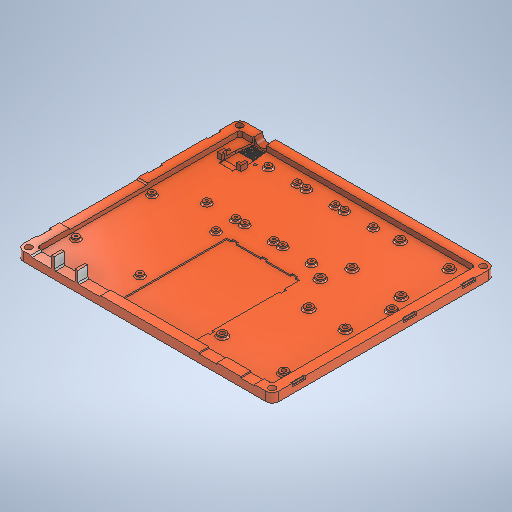
# Autodesk Inventor part: Electronic Base 5
Saved by Autodesk Inventor 2025.2 (Build 292293000, 293)
## iProperties
Created: 2025-02-05
Part Number: Electronic Base 5
Material: Generic
Document SubType Name: Modeling
Designer: caomi
Density: 1 g/cm^3
Appearance: Default
Author: caomi
Autodesk Inventor part; units mm, degrees
ref_plane "YZ Plane" through (0, 0, 0) normal (1, 0, 0) x (0, 1, 0)
ref_plane "XZ Plane" through (0, 0, 0) normal (0, 1, 0) x (-1, 0, 0)
ref_plane "XY Plane" through (0, 0, 0) normal (0, 0, 1) x (1, 0, 0)
sketch "Sketch1" plane through (0, 0, 0) normal (0, 1, 0) x (-1, 0, 0)
  line L0 (195, 170) -> (0, 170)
  line L1 (0, 170) -> (0, 0)
  line L2 (0, 0) -> (195, 0)
  line L3 (195, 0) -> (195, 170)
  line L4 (185.5, 76.5) -> (129.5, 76.5) construction
  line L5 (129.5, 76.5) -> (129.5, 161.5) construction
  line L6 (129.5, 161.5) -> (185.5, 161.5) construction
  line L7 (185.5, 161.5) -> (185.5, 76.5) construction
  circle A0 centre (182, 80) radius 0.9
  circle A1 centre (182, 138) radius 0.9
  circle A2 centre (133, 80) radius 0.9
  circle A3 centre (133, 138) radius 0.9
  line L8 (0, 0) -> (-136.9444, 0) construction
  line L9 (0, 0) -> (0, -49.9102) construction
  circle A4 centre (182, 80) radius 2.4
  circle A5 centre (182, 138) radius 2.4
  circle A6 centre (133, 80) radius 2.4
  circle A7 centre (133, 138) radius 2.4
  line L10 (187.5, 7.5) -> (7.5, 7.5)
  line L11 (7.5, 7.5) -> (7.5, 162.5)
  line L12 (7.5, 162.5) -> (187.5, 162.5)
  line L13 (187.5, 162.5) -> (187.5, 7.5)
  line L14 (64.5, 59.9) -> (11.16, 59.9) construction
  line L15 (11.16, 59.9) -> (11.16, 161.5) construction
  line L16 (11.16, 161.5) -> (64.5, 161.5) construction
  line L17 (64.5, 161.5) -> (64.5, 59.9) construction
  circle A8 centre (61.96, 71.33) radius 3.05
  circle A9 centre (61.96, 71.33) radius 1.55
  circle A10 centre (46.72, 95.46) radius 3.05
  circle A11 centre (46.72, 95.46) radius 1.55
  circle A12 centre (61.96, 146.26) radius 1.55
  circle A13 centre (18.78, 95.46) radius 3.05
  circle A14 centre (61.96, 146.26) radius 3.05
  circle A15 centre (18.78, 95.46) radius 1.55
  circle A16 centre (13.7, 64.98) radius 3.05
  circle A17 centre (13.7, 64.98) radius 1.55
  circle A18 centre (13.7, 147.53) radius 3.05
  circle A19 centre (13.7, 147.53) radius 1.55
  line L18 (124.5, 80.32) -> (69.75, 80.32) construction
  line L19 (69.75, 80.32) -> (69.75, 162) construction
  line L20 (69.75, 162) -> (124.5, 162) construction
  line L21 (124.5, 162) -> (124.5, 80.32) construction
  line L22 (59.33, 12.5) -> (16.33, 12.5) construction
  line L23 (16.33, 12.5) -> (16.33, 55.5) construction
  line L24 (16.33, 55.5) -> (59.33, 55.5) construction
  line L25 (59.33, 55.5) -> (59.33, 12.5) construction
  line L26 (157.5, 66.5) -> (131.5, 66.5) construction
  line L27 (131.5, 66.5) -> (131.5, 15.5) construction
  line L28 (131.5, 15.5) -> (157.5, 15.5) construction
  line L29 (157.5, 15.5) -> (157.5, 66.5) construction
  circle A20 centre (155.5, 17.5) radius 0.9
  circle A21 centre (155.5, 17.5) radius 2.4
  circle A22 centre (133.5, 17.5) radius 2.4
  circle A23 centre (133.5, 17.5) radius 0.9
  circle A24 centre (155.5, 64.5) radius 2.4
  circle A25 centre (155.5, 64.5) radius 0.9
  circle A26 centre (133.5, 64.5) radius 0.9
  circle A27 centre (133.5, 64.5) radius 2.4
  line L30 (102.5, 15.5) -> (128.5, 15.5) construction
  circle A28 centre (104.5, 17.5) radius 0.9
  circle A29 centre (126.5, 17.5) radius 0.9
  circle A30 centre (104.5, 17.5) radius 2.4
  circle A31 centre (126.5, 17.5) radius 2.4
  circle A32 centre (104.5, 64.5) radius 0.9
  circle A33 centre (104.5, 64.5) radius 2.4
  line L31 (102.5, 66.5) -> (102.5, 15.5) construction
  line L32 (128.5, 66.5) -> (102.5, 66.5) construction
  circle A34 centre (126.5, 64.5) radius 2.4
  line L33 (128.5, 15.5) -> (128.5, 66.5) construction
  circle A35 centre (126.5, 64.5) radius 0.9
  line L34 (73.5, 15.5) -> (99.5, 15.5) construction
  circle A36 centre (75.5, 17.5) radius 0.9
  circle A37 centre (97.5, 17.5) radius 0.9
  circle A38 centre (75.5, 17.5) radius 2.4
  circle A39 centre (97.5, 17.5) radius 2.4
  circle A40 centre (75.5, 64.5) radius 0.9
  circle A41 centre (75.5, 64.5) radius 2.4
  line L35 (73.5, 66.5) -> (73.5, 15.5) construction
  line L36 (99.5, 66.5) -> (73.5, 66.5) construction
  circle A42 centre (97.5, 64.5) radius 2.4
  line L37 (99.5, 15.5) -> (99.5, 66.5) construction
  circle A43 centre (97.5, 64.5) radius 0.9
  line L38 (69.25, 79.82) -> (125, 79.82)
  line L39 (125, 79.82) -> (125, 162.5)
  line L40 (125, 162.5) -> (69.25, 162.5)
  line L41 (69.25, 162.5) -> (69.25, 79.82)
  line L42 (99.125, 79.82) -> (95.125, 79.82)
  line L43 (95.125, 79.82) -> (95.125, 78.32)
  line L44 (95.125, 78.32) -> (99.125, 78.32)
  line L45 (99.125, 78.32) -> (99.125, 79.82)
  line L46 (117.825, 78.32) -> (121.825, 78.32)
  line L47 (121.825, 78.32) -> (121.825, 79.82)
  line L48 (117.825, 79.82) -> (117.825, 78.32)
  line L49 (72.425, 78.32) -> (76.425, 78.32)
  line L50 (76.425, 78.32) -> (76.425, 79.82)
  line L51 (72.425, 79.82) -> (72.425, 78.32)
  line L52 (69.25, 146.1) -> (67.75, 146.1)
  line L53 (67.75, 146.1) -> (67.75, 150.1)
  line L54 (67.75, 150.1) -> (69.25, 150.1)
  line L55 (69.25, 150.1) -> (69.25, 146.1)
  line L56 (69.25, 91.57) -> (67.75, 91.57)
  line L57 (67.75, 91.57) -> (67.75, 95.57)
  line L58 (67.75, 95.57) -> (69.25, 95.57)
  circle A44 centre (19.201, 15.82) radius 1.4
  circle A45 centre (19.201, 15.82) radius 2.9
  circle A46 centre (56.574, 15.82) radius 2.9
  circle A47 centre (56.574, 15.82) radius 1.4
  circle A48 centre (19.201, 52.557) radius 1.4
  circle A49 centre (19.201, 52.557) radius 2.9
  circle A50 centre (56.574, 52.557) radius 2.9
  circle A51 centre (56.574, 52.557) radius 1.4
  line L59 (144.5, 15.5) -> (144.5, 27.2667) construction
  line L60 (37.83, 12.5) -> (37.83, 30.4) construction
  line L61 (37.83, 59.9) -> (37.83, 76.07) construction
  point P0 (185.5, 119)
  point P1 (11.16, 110.7)
  point P2 (1.5544, 63)
  point P3 (2.0056, 63)
  point P4 (82.8344, 63)
  point P5 (83.2856, 63)
  point P6 (37.83, 161.5)
  point P7 (97.125, 78.32)
  point P8 (97.125, 79.82)
  point P9 (119.825, 78.32)
  point P10 (74.425, 78.32)
  point P11 (67.75, 148.1)
  point P12 (67.75, 93.57)
  point P13 (72.425, 79.82)
  point P14 (76.425, 79.82)
  point P15 (95.125, 79.82)
  dimension "d10" = 1.8
  dimension "d49" = 53.34
  dimension "d59" = 7.5
  dimension "d62" = 3.1
  dimension "d63" = 1.5
  dimension "d73" = 7.5
  dimension "d79" = 7.5
  dimension "d82" = 2.54
  dimension "d83" = 15.24
  dimension "d84" = 90.17
  dimension "d85" = 96.52
  dimension "d86" = 50.8
  dimension "d87" = 66.04
  dimension "d88" = 17.78
  dimension "d89" = 45.72
  dimension "d90" = 13.97
  dimension "d91" = 85
  dimension "d92" = 58
  dimension "d95" = 1.5
  dimension "d96" = 3.5
  dimension "d97" = 3.5
  dimension "d98" = 3.5
  dimension "d99" = 56
  dimension "d102" = 7.5
  dimension "d103" = 65
  dimension "d121" = 54.75
  dimension "d122" = 81.68
  dimension "d123" = 1
  dimension "d124" = 43
  dimension "d131" = 51
  dimension "d134" = 101.6
  dimension "d135" = 26
  dimension "d141" = 49
  dimension "d144" = 29
  dimension "d149" = 0.5
  dimension "d150" = 4
  dimension "d151" = 1.5
  dimension "d154" = 22.7
  dimension "d160" = 11.9
  dimension "d165" = 54.53
  dimension "d172" = 30
  dimension "d173" = 8
  dimension "d174" = 2
  dimension "d176" = 2.8
  dimension "d178" = 5
  dimension "d179" = 3.32
  dimension "d180" = 2.871
  dimension "d181" = 40.244
  dimension "d182" = 40.057
  dimension "d278" = 1.5
  dimension "d279" = 2
  dimension "d280" = 2
  dimension "d281" = 1.8
  dimension "d282" = 4.8
  dimension "d298" = 155
  dimension "d299" = 4.5
  dimension "d305" = 180
  constraints: 124 end point, 52 centre point, 26 equal radius, 21 coincident, 20 parallel, 13 perpendicular, 12 horizontal, 10 midpoint, 9 vertical alignment, 7 horizontal alignment, 5 vertical, 4 collinear, 3 point on line, 1 symmetric about line, 74 other
  measures "d10" diameter of A0
  measures "d49" distance of L15.end L16.end
  measures "d59" distance between parallel lines of L13 L3
  measures "d62" diameter of A9
  measures "d63" radial gap between concentric circles of A8 A9
  measures "d73" distance between parallel lines of L0 L12
  measures "d79" distance between parallel lines of L2 L10
  measures "d82" distance from line of L17 A12.centre
  measures "d83" distance from line of L16 A12.centre
  measures "d84" distance from line of L16 A9.centre
  measures "d85" distance from line of L16 A16.centre
  measures "d86" distance from line of L17 A17.centre
  measures "d87" distance from line of L16 A10.centre
  measures "d88" distance from line of L17 A10.centre
  measures "d89" distance from line of L17 A15.centre
  measures "d90" distance from line of L16 A18.centre
  measures "d91" distance of L4.end L5.end
  measures "d92" distance of A3.centre A2.centre
  measures "d95" radial gap between concentric circles of A4 A0
  measures "d96" distance from line of L4 A2.centre
  measures "d97" distance from line of L7 A0.centre
  measures "d98" distance from line of L5 A2.centre
  measures "d99" distance between parallel lines of L7 L5
  measures "d102" distance between parallel lines of L1 L11
  measures "d103" distance between parallel lines of L17 L5
  measures "d121" distance of L19.end L20.end
  measures "d122" distance of L18.end L19.end
  measures "d123" distance between parallel lines of L12 L16
  measures "d124" distance of L22.end L23.end
  measures "d131" distance of L28.end L26.start
  measures "d134" distance of L14.end L15.end
  measures "d135" distance of L27.end L28.end
  measures "d141" distance from line of L28 A24.centre
  measures "d144" distance of A22.centre A30.centre
  measures "d149" distance between parallel lines of L19 L41
  measures "d150" distance of L43.end L44.end
  measures "d151" distance between parallel lines of L38 L44
  measures "d154" distance of point (97.125, 78.32) point (119.825, 78.32)
  measures "d160" distance between parallel lines of L20 L54
  measures "d165" distance of L52.start L56.start
  measures "d172" distance between parallel lines of L13 L29
  measures "d173" distance between parallel lines of L10 L28
  measures "d174" distance between parallel lines of L7 L13
  measures "d176" diameter of A44
  measures "d178" vertical distance of L10.end L22.end
  measures "d179" distance from line of L22 A44.centre
  measures "d180" distance from line of L23 A44.centre
  measures "d181" distance from line of L23 A46.centre
  measures "d182" distance from line of L22 A48.centre
  measures "d278" radial gap between concentric circles of A44 A45
  measures "d279" distance from line of A21.centre L29
  measures "d280" distance from line of A20.centre L28
  measures "d281" diameter of A20
  measures "d282" diameter of A21
  measures "d298" distance of L10.end L11.end
  measures "d299" distance between parallel lines of L5 L39
  measures "d305" distance of L11.end L12.end
extrude "Base" add sketch "Sketch1" against normal blind 3 contours L3 L2 L1 L0 | A0 | A1 | A2 | A3 | A4 | A5 | A6 | A7 | L10 L11 L12 L41 L54 L53 L52 L58 L57 L56 L38 L51 L49 L50 L43 L44 L45 L48 L46 L47 L39 L13 | L39 L38 L41 L12 | L41 L52 L53 L54 | L47 L46 L48 L38 | L41 L56 L57 L58 | L45 L44 L43 L38 | L50 L49 L51 L38 | A8 | A9 | A10 | A11 | A12 | A13 | A14 | A15 | A16 | A17 | A18 | A19 | A20 | A21 | A22 | A23 | A24 | A25 | A26 | A27 | A28 | A29 | A30 | A31 | A32 | A33 | A34 | A35 | A36 | A37 | A38 | A39 | A40 | A41 | A42 | A43 | A44 | A45 | A46 | A47 | A48 | A49 | A50 | A51
extrude "Wall" add sketch "Sketch1" along normal blind 4 contours L3 L2 L1 L0
extrude "Breadboard Slot" cut sketch "Sketch1" against normal blind 1 contours L39 L38 L41 L12 | L41 L52 L53 L54 | L47 L46 L48 L38 | L41 L56 L57 L58 | L45 L44 L43 L38 | L50 L49 L51 L38
extrude "Electronic Mounting Holes" add sketch "Sketch1" along normal blind 2 contours A4 | A5 | A6 | A7 | A8 | A10 | A13 | A14 | A16 | A18 | A21 | A22 | A24 | A27 | A30 | A31 | A33 | A34 | A38 | A39 | A41 | A42 | A45 | A46 | A49 | A50
extrude "Deeper Mounting Holes" cut sketch "Sketch1" against normal blind 2 contours A0 | A1 | A2 | A3 | A9 | A11 | A12 | A15 | A17 | A19 | A20 | A23 | A25 | A26 | A28 | A29 | A32 | A35 | A36 | A37 | A40 | A43 | A44 | A47 | A48 | A51
chamfer "Chamfer2" distance 1 angle 45 26 edges at (-153.1, 0, 17.5) (-131.1, 0, 17.5) (-124.1, 0, 17.5) (-102.1, 0, 17.5) (-95.1, 0, 17.5) (-73.1, 0, 17.5) (-53.674, 0, 15.82) (-16.301, 0, 15.82) (-16.301, 0, 52.557) (-10.65, 0, 64.98) (-53.674, 0, 52.557) (-58.91, 0, 71.33) (-73.1, 0, 64.5) (-95.1, 0, 64.5) (-102.1, 0, 64.5) (-124.1, 0, 64.5) (-131.1, 0, 64.5) (-153.1, 0, 64.5) (-130.6, 0, 80) (-179.6, 0, 80) (-179.6, 0, 138) (-130.6, 0, 138) (-43.67, 0, 95.46) (-15.73, 0, 95.46) (-10.65, 0, 147.53) (-58.91, 0, 146.26)
fillet "Fillet1" radius 5 4 edges at (-195, 0.5, 0) (0, 0.5, 170) (-195, 0.5, 170) (0, 0.5, 0)
fillet "Fillet3" radius 2 4 edges at (-187.5, 2, 162.5) (-187.5, 2, 7.5) (-7.5, 2, 162.5) (-7.5, 2, 7.5)
sketch "Sketch2" plane through (0, 4, 0) normal (0, 1, 0) x (1, 0, 0)
  line L0 (-190, -170) -> (-5, -170) projected
  line L1 (-7.5, -162.5) -> (-187.5, -162.5) projected
  line L2 (-184.5, -162.5) -> (-168.5, -162.5)
  line L3 (-168.5, -162.5) -> (-168.5, -170)
  line L4 (-168.5, -170) -> (-184.5, -170)
  line L5 (-184.5, -170) -> (-184.5, -162.5)
  line L6 (-166.5, -162.5) -> (-150.5, -162.5)
  line L7 (-150.5, -162.5) -> (-150.5, -170)
  line L8 (-150.5, -170) -> (-166.5, -170)
  line L9 (-166.5, -170) -> (-166.5, -162.5)
  line L10 (-148.5, -162.5) -> (-131, -162.5)
  line L11 (-131, -162.5) -> (-131, -170)
  line L12 (-131, -170) -> (-148.5, -170)
  line L13 (-148.5, -170) -> (-148.5, -162.5)
  line L14 (-56, -162.5) -> (-42.36, -162.5)
  line L15 (-42.36, -162.5) -> (-42.36, -170)
  line L16 (-42.36, -170) -> (-56, -170)
  line L17 (-56, -170) -> (-56, -162.5)
  line L18 (-185.5, -161.5) -> (-185.5, -76.5) construction
  line L19 (-64.5, -161.5) -> (-64.5, -59.9) construction
  line L20 (-24, -162.5) -> (-13.67, -162.5)
  line L21 (-13.67, -162.5) -> (-13.67, -170)
  line L22 (-13.67, -170) -> (-24, -170)
  line L23 (-24, -170) -> (-24, -162.5)
  line L24 (-195, -5) -> (-195, -165) projected
  line L25 (-187.5, -9.5) -> (-187.5, -160.5) projected
  line L26 (-195, -137.5) -> (-187.5, -137.5)
  line L27 (-187.5, -137.5) -> (-187.5, -77.5)
  line L28 (-187.5, -77.5) -> (-195, -77.5)
  line L29 (-195, -77.5) -> (-195, -137.5)
  point P0 (0, 0)
  point P1 (-150.5, -162.5)
  point P2 (-168.5, -162.5)
  point P3 (-13.67, -166.25)
  point P4 (-56, -170)
  point P5 (-195, -77.5)
  point P6 (-187.5, -137.5)
  dimension "d104" = 16
  dimension "d107" = 16
  dimension "d109" = 17.5
  dimension "d113" = 13.64
  dimension "d114" = 1
  dimension "d115" = 19
  dimension "d116" = 37
  dimension "d117" = 8.5
  dimension "d118" = 40.5
  dimension "d119" = 10.33
  dimension "d300" = 25
  dimension "d301" = 85
  constraints: 48 end point, 12 parallel, 12 point on line, 6 horizontal, 6 perpendicular, 1 midpoint
  measures "d104" distance of L3.end L4.end
  measures "d107" distance of L7.end L8.end
  measures "d109" distance between parallel lines of L11 L13
  measures "d113" distance between parallel lines of L15 L17
  measures "d114" distance between parallel lines of L18 L5
  measures "d115" distance between parallel lines of L18 L9
  measures "d116" distance between parallel lines of L18 L13
  measures "d117" distance between parallel lines of L19 L17
  measures "d118" distance between parallel lines of L19 L23
  measures "d119" distance from line of point (-13.67, -166.25) L23
  measures "d300" vertical distance of L1.end L26.start
  measures "d301" vertical distance of L1.end L28.end
extrude "Board ports" cut sketch "Sketch2" against normal blind 1 contours L5 L1 L3 L0 | L9 L1 L7 L0 | L13 L1 L11 L0 | L17 L1 L15 L0 | L23 L1 L21 L0 | L28 L25 L26 L24
chamfer "Chamfer3" distance 1 angle 45 6 edges at (-184.5, 3, 166.25) (-168.5, 3, 166.25) (-166.5, 3, 166.25) (-150.5, 3, 166.25) (-148.5, 3, 166.25) (-131, 3, 166.25)
extrude "Extrusion18" add sketch "Sketch2" along normal blind 8 contours L3 L1 L9 L0 | L7 L1 L13 L0
fillet "Fillet5" radius 1 2 edges at (-191.25, 3, 77.5) (-191.25, 3, 137.5)
sketch "Sketch3" plane through (-188.34, 0, 170) normal (0, 0, 1) x (1, 0, 0)
  line L0 (-4.66, 2.5) -> (-5.66, 1.5)
  line L1 (-4.66, 2.5) -> (-5.66, 3.5)
  line L2 (-4.66, 2.5) -> (-5.66, 2.5) construction
  line L3 (-6.66, -3) -> (-6.66, 4) projected
  line L4 (-6.66, 4) -> (-5.66, 4)
  line L5 (-5.66, 4) -> (-5.66, 1.5)
  line L6 (-5.66, 1.5) -> (-6.66, 1.5)
  line L7 (-6.66, 1.5) -> (-6.66, 4)
  point P0 (188.34, 0)
  point P1 (-4, 3.1514)
  dimension "d201" = 1
  dimension "d210" = 2.5
  dimension "d211" = 1
  dimension "d222" = 45
  constraints: 14 end point, 2 horizontal, 2 parallel, 2 point on line, 1 perpendicular, 1 other
  measures "d201" distance of L0.start L2.end
  measures "d210" distance between parallel lines of L4 L6
  measures "d211" distance of L3.end L4.end
  measures "d222" angle of L0 L5
ref_plane "Work Plane6" through (-190, -3, 150) normal (0, 0, 1) x (1, 0, 0)
ref_plane "Work Plane7" through (-190, -3, 65) normal (0, 0, 1) x (1, 0, 0)
ref_plane "Work Plane8" through (-190, -3, 20) normal (0, 0, 1) x (1, 0, 0)
extrude "Extrusion6" cut sketch "Sketch3" along normal mid plane 10 from surface at -20
extrude "Extrusion16" cut sketch "Sketch3" along normal mid plane 10 from surface at -105
extrude "Extrusion17" cut sketch "Sketch3" along normal mid plane 10 from surface at -150
fillet "Fillet4" radius 1 3 edges at (-193, 2.5, 150) (-193, 2.5, 65) (-193, 2.5, 20)
ref_plane "Work Plane3" through (-97.5, -3, 5) normal (1, 0, 0) x (0, 0, -1)
mirror "Mirror2" about plane through (-97.5, -3, 5) normal (1, 0, 0) of "Extrusion6", "Extrusion16", "Extrusion17", "Fillet4"
sketch "Sketch4" plane through (0, 4, 0) normal (0, 1, 0) x (1, 0, 0)
  line L0 (-192.1454, -1.65) -> (-188.8546, -1.65)
  line L1 (-188.8546, -1.65) -> (-187.2091, -4.5)
  line L2 (-187.2091, -4.5) -> (-188.8546, -7.35)
  line L3 (-188.8546, -7.35) -> (-192.1454, -7.35)
  line L4 (-192.1454, -7.35) -> (-193.7909, -4.5)
  line L5 (-193.7909, -4.5) -> (-192.1454, -1.65)
  line L6 (-195, -5) -> (-195, -165) projected
  line L7 (-5, 0) -> (-190, 0) projected
  point P0 (0, 0)
  point P1 (-190.5, -4.5)
  point P2 (-193.34, -28.8)
  dimension "d205" = 5.7
  dimension "d206" = 4.5
  dimension "d207" = 4.5
  constraints: 12 end point, 1 horizontal, 14 other
  measures "d205" distance between parallel lines of L0 L3
  measures "d207" distance from line of L7 point (-190.5, -4.5)
extrude "Extrusion7" cut sketch "Sketch4" along normal blind 1 from surface at -7
hole "Hole1" at (-190.5, 4, 4.5) direction (0, -1, 0) diameter 3 end through all counterbore diameter 5 counterbore depth 3.2
mirror "Mirror3" about plane through (-97.5, -3, 5) normal (1, 0, 0) of "Hole1", "Extrusion7"
ref_plane "Work Plane9" through (-5, -3, 85) normal (0, 0, -1) x (-1, 0, 0)
mirror "Mirror5" about plane through (-5, -3, 85) normal (0, 0, -1) of "Hole1", "Extrusion7", "Mirror3"
sketch "Sketch6" plane through (0, 4, 0) normal (0, 1, 0) x (1, 0, 0)
  line L0 (-177.75, -6) -> (-167.25, -6)
  line L1 (-167.25, -6) -> (-165.5, -19)
  line L2 (-179.5, -19) -> (-177.75, -6)
  line L3 (-172.5, 8.2313) -> (-172.5, -20.9811) construction
  line L4 (-167.0346, -7.6) -> (-177.9654, -7.6)
  line L5 (-166.9269, -8.4) -> (-178.0731, -8.4)
  line L6 (-166.7654, -9.6) -> (-178.2346, -9.6)
  line L7 (-166.6577, -10.4) -> (-178.3423, -10.4)
  line L8 (-166.4962, -11.6) -> (-178.5038, -11.6)
  line L9 (-166.3885, -12.4) -> (-178.6115, -12.4)
  line L10 (-166.2269, -13.6) -> (-178.7731, -13.6)
  line L11 (-165.85, -16.4) -> (-179.15, -16.4)
  line L12 (-165.9577, -15.6) -> (-179.0423, -15.6)
  line L13 (-165.5, -19) -> (-165.5, -28.5)
  line L14 (-179.5, -28.5) -> (-179.5, -19)
  line L15 (-5, 0) -> (-190, 0) projected
  line L16 (-166.1192, -14.4) -> (-178.8808, -14.4)
  line L17 (-167.25, -28.5) -> (-167.25, -33)
  line L18 (-167.25, -33) -> (-177.75, -33)
  line L19 (-177.75, -33) -> (-177.75, -28.5)
  line L20 (-165.6885, -17.6) -> (-179.3115, -17.6)
  line L21 (-165.5808, -18.4) -> (-179.4192, -18.4)
  line L22 (-165.5, -28.5) -> (-167.25, -28.5)
  line L23 (-177.75, -28.5) -> (-179.5, -28.5)
  line L24 (-177.75, -28.5) -> (-167.25, -28.5)
  line L25 (-179.5, -25.5) -> (-181.5, -25.5)
  line L26 (-181.5, -25.5) -> (-181.5, -30.5)
  line L27 (-181.5, -30.5) -> (-178, -30.5)
  line L28 (-178, -30.5) -> (-178, -28.5)
  line L29 (-165.5, -25.5) -> (-163.5, -25.5)
  line L30 (-163.5, -25.5) -> (-163.5, -30.5)
  line L31 (-163.5, -30.5) -> (-167, -30.5)
  line L32 (-167, -30.5) -> (-167, -28.5)
  line L33 (-187.5, -160.5) -> (-187.5, -9.5) projected
  point P0 (0, -28.8)
  point P1 (-165.5, -25.5)
  dimension "d223" = 10.5
  dimension "d224" = 14
  dimension "d226" = 1.6
  dimension "d227" = 0.8
  dimension "d228" = 1.2
  dimension "d229" = 0.8
  dimension "d230" = 1.2
  dimension "d231" = 0.8
  dimension "d232" = 1.2
  dimension "d235" = 0.8
  dimension "d240" = 6
  dimension "d241" = 0.8
  dimension "d242" = 1.2
  dimension "d253" = 10.5
  dimension "d255" = 1.2
  dimension "d260" = 0.8
  dimension "d261" = 13
  dimension "d262" = 9.5
  dimension "d263" = 4.5
  dimension "d265" = 2
  dimension "d266" = 2
  dimension "d267" = 3
  dimension "d268" = 1.5
  dimension "d297" = 15
  constraints: 60 end point, 18 horizontal, 5 symmetric about line, 2 parallel, 2 perpendicular, 2 point on line, 2 vertical, 1 collinear, 32 other
  measures "d223" distance of L0.start L0.end
  measures "d224" distance of L14.end L13.start
  measures "d226" distance between parallel lines of L4 L0
  measures "d227" distance between parallel lines of L5 L4
  measures "d228" distance between parallel lines of L5 L6
  measures "d229" distance between parallel lines of L6 L7
  measures "d230" distance between parallel lines of L8 L7
  measures "d231" distance between parallel lines of L8 L9
  measures "d232" distance between parallel lines of L10 L9
  measures "d235" distance between parallel lines of L12 L11
  measures "d240" distance between parallel lines of L15 L0
  measures "d241" distance between parallel lines of L10 L16
  measures "d242" distance between parallel lines of L16 L12
  measures "d253" distance of L17.end L18.end
  measures "d255" distance between parallel lines of L20 L11
  measures "d260" distance between parallel lines of L20 L21
  measures "d261" vertical distance of L13.start L0.end
  measures "d262" distance of L13.start L13.end
  measures "d263" distance between parallel lines of L22 L18
  measures "d265" distance of L27.end L28.end
  measures "d266" distance of L25.start L25.end
  measures "d267" distance between parallel lines of L23 L25
  measures "d268" distance between parallel lines of L28 L14
  measures "d297" distance between parallel lines of L33 L3
extrude "DC terminal slot" cut sketch "Sketch6" against normal blind 6 contours L0 L1 L4 L2 | L4 L1 L5 L2 | L5 L1 L6 L2 | L6 L1 L7 L2 | L7 L1 L8 L2 | L8 L1 L9 L2 | L9 L1 L10 L2 | L10 L1 L16 L2 | L16 L1 L12 L2 | L12 L1 L11 L2 | L11 L1 L20 L2 | L20 L1 L21 L2 | L21 L1 L13 L22 L24 L23 L14 L2 | L24 L17 L18 L19
extrude "DC terminal ribs" add sketch "Sketch6" along normal blind 0.5 from surface at -6 contours L4 L1 L5 L2 | L6 L1 L7 L2 | L8 L1 L9 L2 | L10 L1 L16 L2 | L12 L1 L11 L2
extrude "DC terminal output" add sketch "Sketch6" along normal blind 1 from surface at -5.5 contours L24 L17 L18 L19
sketch "Sketch7" plane through (-177.75, 4, 6) normal (0, 0, 1) x (1, 0, 0)
  circle A0 centre (5.25, 0) radius 5
  line L0 (0, -6) -> (10.5, -6) projected
  point P0 (177.75, -4)
  point P1 (5.25, -6)
  point P2 (5.25, -6)
  dimension "d249" = 6
  dimension "d250" = 10
  constraints: 2 midpoint, 1 centre point, 1 vertical alignment
  measures "d249" distance of point (5.25, -6) A0.centre
  measures "d250" diameter of A0
extrude "DC terminal port" cut sketch "Sketch7" against normal up to surface (6 mm away)
extrude "Extrusion13" add sketch "Sketch6" against normal up to surface (4 mm away) contours L14 L23 L28 L27 L26 L25 | L29 L30 L31 L32 L22 L13
sketch "Sketch8" plane through (0, 4, 0) normal (0, 1, 0) x (1, 0, 0)
  line L0 (-190, 0) -> (-5, 0) projected
  line L1 (-185, 0) -> (-160, 0)
  line L2 (-160, 0) -> (-160, -35)
  line L3 (-160, -35) -> (-185, -35)
  line L4 (-185, -35) -> (-185, 0)
  line L5 (-172.5, 8.2313) -> (-172.5, -20.9811) construction
  point P0 (0, 0)
  point P1 (-160, 0)
  dimension "d256" = 25
  dimension "d257" = 35
  constraints: 8 end point, 2 parallel, 1 horizontal, 1 perpendicular, 1 point on line, 1 other
  measures "d256" distance between parallel lines of L4 L2
  measures "d257" distance of L1.end L2.end
extrude "DC Jack Test Fit" [suppressed]
sketch "Sketch9" plane through (0, 0, 0) normal (0, 1, 0) x (1, 0, 0)
  circle A0 centre (-182.5, -20.5) radius 1
  circle A1 centre (-162.5, -20.5) radius 1
  line L0 (-172.5, 8.2313) -> (-172.5, -20.9811) construction
  line L1 (-167.25, -28.5) -> (-177.75, -28.5) projected
  point P0 (0, 0)
  dimension "d272" = 20
  dimension "d273" = 2
  dimension "d274" = 8
  constraints: 2 centre point, 1 equal radius, 1 horizontal alignment, 1 other
  measures "d272" distance of A0.centre A1.centre
  measures "d273" diameter of A0
  measures "d274" distance from line of L1 A0.centre
extrude "Extrusion14" cut sketch "Sketch9" against normal blind 10
ref_plane "Work Plane4" through (-97.5, -3, 5) normal (1, 0, 0) x (0, 0, -1)
equation "\"board_border\" = 2"
equation "\"base_wall\" = 7.5"
body "Solid1"
